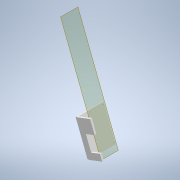
# Autodesk Inventor part: servo_mount
Saved by Autodesk Inventor 2021 (Build 250183000, 183)
## iProperties
Created: 2021-11-19
Part Number: servo_mount
Material: Generic
Document SubType Name: Modeling
Designer: techv
Density: 1 g/cm^3
Appearance: Default
Author: techv
Autodesk Inventor part; units mm, degrees
ref_plane "YZ Plane" through (0, 0, 0) normal (1, 0, 0) x (0, 1, 0)
ref_plane "XZ Plane" through (0, 0, 0) normal (0, 1, 0) x (-1, 0, 0)
ref_plane "Work Plane1" through (-95.5841, -36.463, 65.2713) normal (-0.9323109, -0.3616579, 0) x (0.3616579, -0.9323109, 0)
sketch "Sketch1" plane through (-95.5841, -36.463, 65.2713) normal (-0.9323109, -0.3616579, 0) x (0.3616579, -0.9323109, 0)
  arc A0 (-290.5, 45) -> (-292.5, 43) centre (-290.5, 43) ccw projected
  line L0 (-292.5, 1) -> (-292.5, 43) projected
  line L1 (-10, 1) -> (-292.5, 1) projected
  line L2 (-10, 1) -> (-10, 43) projected
  arc A1 (-10, 43) -> (-12, 45) centre (-12, 43) ccw projected
  line L3 (-12, 45) -> (-290.5, 45) projected
  circle A2 centre (-205.5, 4.5) radius 1.4 projected
  circle A3 centre (-288.25, 40.5) radius 1.4 projected
  circle A4 centre (-288.25, 4.5) radius 1.4 projected
  circle A5 centre (-97, 40.5) radius 1.4 projected
  circle A6 centre (-97, 4.5) radius 1.4 projected
  circle A7 centre (-14.25, 40.5) radius 1.4 projected
  circle A8 centre (-14.25, 4.5) radius 1.4 projected
  circle A9 centre (-205.5, 40.5) radius 1.4 projected
  line L4 (-73.16, 76.2) -> (-67.3719, 76.2) projected
  line L5 (-118.5085, 48.1443) -> (-185.5357, 48.1443) projected
  line L6 (-10, 1) -> (-102.3549, 1)
  line L7 (-102.3549, 1) -> (-102.3549, 74.6175)
  line L8 (-102.3549, 74.6175) -> (-10, 74.6175)
  line L9 (-10, 74.6175) -> (-10, 1)
  point P0 (0.5739, -65.2713)
  point P1 (-102.3549, 1)
  point P2 (-10, 43)
  constraints: 8 end point, 2 parallel, 1 horizontal, 1 perpendicular
extrude "Extrusion1" add sketch "Sketch1" along normal blind 5 contours L7 L8 L9 A1 L3 | L3 A1 L2 L1 L7
sketch "Sketch2" plane through (-95.5841, -36.463, 65.2713) normal (0.9323109, 0.3616579, 0) x (0, 0, -1)
  line L0 (-76.2, 21.2) -> (-76.2, 20.15) projected
  line L1 (-1, 10) -> (-74.6175, 10) projected
  line L2 (-74.6175, 102.3549) -> (-1, 102.3549) projected
  line L3 (-76.2, 10) -> (-71.2, 10)
  line L4 (-71.2, 10) -> (-71.2, 102.3549)
  line L5 (-71.2, 102.3549) -> (-76.2, 102.3549)
  line L6 (-76.2, 102.3549) -> (-76.2, 10)
  line L7 (-76.08, 27) -> (-70.4, 27) projected
  line L8 (-70.4, 67.36) -> (-76.08, 67.36) projected
  line L9 (-71.2, 27) -> (-76.08, 27)
  line L10 (-71.2, 67.36) -> (-76.2, 67.36)
  line L11 (-76.0598, 27) -> (-76.2, 27)
  line L12 (-76.0598, 27) -> (-75.9197, 27) construction
  point P0 (65.2713, -0.5739)
  point P1 (-76.08, 67.36)
  point P2 (-76.2, 21.2)
  point P3 (-76.2, 20.15)
  dimension "d2" = 5
  dimension "d3" = 180
  constraints: 16 end point, 10 point on line, 2 collinear, 2 horizontal, 2 parallel, 2 perpendicular
  measures "d2" distance of L5.end L4.end
  measures "d3" angle of L11 L12
extrude "Extrusion2" add sketch "Sketch2" along normal blind 40 contours L6 L11 L7 L4 L1 L3 L0 | L6 L5 L2 L4 L8 L10
sketch "Sketch3" plane through (-95.5841, -36.463, 65.2713) normal (0.9323109, 0.3616579, 0) x (0, 0, -1)
  line L0 (-76.2, 102.3549) -> (-76.2, 67.36) projected
  line L1 (-76.2, 27) -> (-76.2, 10) projected
  line L2 (-71.2, 10) -> (-71.2, 27) projected
  line L3 (-76.2, 67.36) -> (-70.5815, 67.36)
  line L4 (-70.5815, 67.36) -> (-70.5815, 27)
  line L5 (-70.5815, 27) -> (-76.2, 27)
  line L6 (-76.2, 27) -> (-76.2, 67.36)
  point P0 (65.2713, -0.5739)
  constraints: 8 end point, 2 parallel, 1 horizontal, 1 perpendicular
ref_plane "Work Plane2" through (-92.6568, -5.2986, 135.4694) normal (-0.9323109, -0.3616579, 0) x (0, 0, 1)
extrude "Extrusion3" add sketch "Sketch3" along normal up to surface (14 mm away)
draft "FaceDraft1" angle 2.5 pull direction (0, 0, 1) faces at (-125.3345, 26.4048, 128.7331) fixed edges at (-120.5627, 14.1036, 139.8888)
sketch "Sketch4" plane through (-95.5841, -36.463, 65.2713) normal (-0.9323109, -0.3616579, 0) x (0, 0, 1)
  line L0 (74.6175, 10) -> (74.6175, 102.3549) projected
  line L1 (76.2, 102.3549) -> (76.2, 10) projected
  line L2 (74.6175, 102.3549) -> (76.2, 102.3549)
  line L3 (76.2, 102.3549) -> (76.2, 10)
  line L4 (76.2, 10) -> (74.6175, 10)
  line L5 (74.6175, 10) -> (74.6175, 102.3549)
  point P0 (-65.2713, -0.5739)
  point P1 (74.6175, 10)
  constraints: 8 end point, 2 parallel, 1 horizontal, 1 perpendicular
extrude "Extrusion4" add sketch "Sketch4" along normal up to surface surface through (-122.0596, 13.5229, 103.1151) normal (-0.9314235, -0.3613137, 0.0436194)
sketch "Sketch5" plane through (-82.653, 40.8038, 141.4713) normal (0, 0, 1) x (0.9323109, 0.3616579, 0)
  arc A0 (-9.1421, -45.9774) -> (-11.7079, -45.9774) centre (-10.425, -44.135) ccw projected
  arc A1 (-20.305, -46.0225) -> (-21.575, -41.86) centre (-21.575, -44.135) ccw projected
  arc A2 (-21.575, -41.86) -> (-22.845, -46.0225) centre (-21.575, -44.135) ccw projected
  arc A3 (-22.8579, 5.6174) -> (-20.2921, 5.6174) centre (-21.575, 3.775) ccw projected
  arc A4 (-11.7079, 5.6174) -> (-9.1421, 5.6174) centre (-10.425, 3.775) ccw projected
  circle A5 centre (-10.425, -44.135) radius 2.245
  circle A6 centre (-21.575, -44.135) radius 2.275
  circle A7 centre (-21.575, 3.775) radius 2.245
  circle A8 centre (-10.425, 3.775) radius 2.245
  point P0 (62.3013, -67.9339)
  point P1 (-22.8579, 5.6174)
  point P2 (-11.7079, 5.6174)
  point P3 (-19.5059, -45.0808)
  point P4 (-9.1421, -45.9774)
  constraints: 4 coincident, 12 other
extrude "Extrusion5" cut sketch "Sketch5" against normal through all
sketch "Sketch6" plane through (-99.2007, -27.1399, 66.2713) normal (0.3616579, -0.9323109, 0) x (0.9323109, 0.3616579, 0)
  line L0 (0, 0) -> (-5, 0)
  line L1 (-5, 0) -> (-5, 75.203)
  line L2 (-5, 75.203) -> (0, 75.203)
  line L3 (0, 75.203) -> (0, 0)
  line L4 (0, 0) -> (-8.2142, 0) projected
  line L5 (-8.2142, 0) -> (-4.9309, 75.2) projected
  point P0 (102.3013, -66.2713)
  point P1 (-5, 73.6175)
  dimension "d13" = 5
  constraints: 8 end point, 2 parallel, 1 horizontal, 1 perpendicular
  measures "d13" distance of L1.end L2.end
extrude "Extrusion6" cut sketch "Sketch6" against normal through all contours L4 L5 L1
fillet "Fillet1" radius 5 4 edges at (-120.4983, 14.1286, 141.4713) (-126.2735, 42.6505, 136.4713) (-102.2748, -19.2152, 136.4713) (-120.5627, 14.1036, 139.8888)
body "Solid1"
